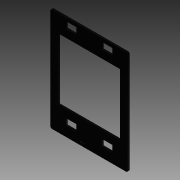
# Autodesk Inventor part: BED HOT BED INSET
Saved by Autodesk Inventor 2013 (Build 170138000, 138)
## iProperties
Created: 2014-03-03
Part Number: BED HOT BED INSET
Material: Generic
Document SubType Name: Modeling
Designer: employee
Density: 1 g/cm^3
Author: employee
Autodesk Inventor part; units mm, degrees
ref_plane "YZ Plane" through (0, 0, 0) normal (1, 0, 0) x (0, 1, 0)
ref_plane "XZ Plane" through (0, 0, 0) normal (0, 1, 0) x (-1, 0, 0)
ref_plane "XY Plane" through (0, 0, 0) normal (0, 0, 1) x (1, 0, 0)
sketch "Sketch1" plane through (0, 0, 0) normal (0, 0, 1) x (1, 0, 0)
  arc A0 (127, -140) -> (122, -135) centre (122, -140) ccw projected
  line L0 (122, -135) -> (119.8284, -135) projected
  line L1 (119.8284, -135) -> (119.8284, -145) projected
  line L2 (119.8284, -145) -> (114.1716, -145) projected
  line L3 (114.1716, -145) -> (114.1716, -135) projected
  line L4 (114.1716, -135) -> (109.5, -135) projected
  arc A1 (107, -132.5) -> (109.5, -135) centre (109.5, -132.5) ccw projected
  line L5 (107, -132.5) -> (107, 132.5) projected
  arc A2 (109.5, 135) -> (107, 132.5) centre (109.5, 132.5) ccw projected
  line L6 (109.5, 135) -> (114.1716, 135) projected
  line L7 (114.1716, 135) -> (114.1716, 145) projected
  line L8 (114.1716, 145) -> (119.8284, 145) projected
  line L9 (119.8284, 145) -> (119.8284, 135) projected
  line L10 (119.8284, 135) -> (122, 135) projected
  arc A3 (122, 135) -> (127, 140) centre (122, 140) ccw projected
  line L11 (127, 140) -> (127, 165) projected
  arc A4 (127, 165) -> (122, 170) centre (122, 165) ccw projected
  line L12 (122, 170) -> (-122, 170) projected
  arc A5 (-122, 170) -> (-127, 165) centre (-122, 165) ccw projected
  line L13 (-127, 165) -> (-127, 140) projected
  arc A6 (-127, 140) -> (-122, 135) centre (-122, 140) ccw projected
  line L14 (-122, 135) -> (-119.8284, 135) projected
  line L15 (-119.8284, 135) -> (-119.8284, 145) projected
  line L16 (-119.8284, 145) -> (-114.1716, 145) projected
  line L17 (-114.1716, 145) -> (-114.1716, 135) projected
  line L18 (-114.1716, 135) -> (-109.5, 135) projected
  arc A7 (-107, 132.5) -> (-109.5, 135) centre (-109.5, 132.5) ccw projected
  line L19 (-107, 132.5) -> (-107, -132.5) projected
  arc A8 (-109.5, -135) -> (-107, -132.5) centre (-109.5, -132.5) ccw projected
  line L20 (-109.5, -135) -> (-114.1716, -135) projected
  line L21 (-114.1716, -135) -> (-114.1716, -145) projected
  line L22 (-114.1716, -145) -> (-119.8284, -145) projected
  line L23 (-119.8284, -145) -> (-119.8284, -135) projected
  line L24 (-119.8284, -135) -> (-122, -135) projected
  arc A9 (-122, -135) -> (-127, -140) centre (-122, -140) ccw projected
  line L25 (-127, -140) -> (-127, -165) projected
  arc A10 (-127, -165) -> (-122, -170) centre (-122, -165) ccw projected
  line L26 (-122, -170) -> (122, -170) projected
  arc A11 (122, -170) -> (127, -165) centre (122, -165) ccw projected
  line L27 (127, -165) -> (127, -140) projected
  line L28 (113, -142) -> (112, -142) projected
  line L29 (112, -142) -> (112, -138) projected
  line L30 (112, -138) -> (113, -138) projected
  line L31 (113, -138) -> (113, -142) projected
  line L32 (121, -142) -> (121, -138) projected
  line L33 (121, -138) -> (122, -138) projected
  line L34 (122, -138) -> (122, -142) projected
  line L35 (122, -142) -> (121, -142) projected
  line L36 (-112, -142) -> (-113, -142) projected
  line L37 (-113, -142) -> (-113, -138) projected
  line L38 (-113, -138) -> (-112, -138) projected
  line L39 (-112, -138) -> (-112, -142) projected
  line L40 (-121, -138) -> (-121, -142) projected
  line L41 (-121, -142) -> (-122, -142) projected
  line L42 (-122, -142) -> (-122, -138) projected
  line L43 (-122, -138) -> (-121, -138) projected
  line L44 (112, 142) -> (113, 142) projected
  line L45 (113, 142) -> (113, 138) projected
  line L46 (113, 138) -> (112, 138) projected
  line L47 (112, 138) -> (112, 142) projected
  line L48 (121, 138) -> (121, 142) projected
  line L49 (121, 142) -> (122, 142) projected
  line L50 (122, 142) -> (122, 138) projected
  line L51 (122, 138) -> (121, 138) projected
  line L52 (-122, 138) -> (-122, 142) projected
  line L53 (-122, 142) -> (-121, 142) projected
  line L54 (-121, 142) -> (-121, 138) projected
  line L55 (-121, 138) -> (-122, 138) projected
  line L56 (-112, 142) -> (-112, 138) projected
  line L57 (-112, 138) -> (-113, 138) projected
  line L58 (-113, 138) -> (-113, 142) projected
  line L59 (-113, 142) -> (-112, 142) projected
  line L60 (-127, 140) -> (-127, -140)
  line L61 (127, -140) -> (127, 140)
  arc A12 (20.5, 83.5) -> (-1.5, 83.5) centre (9.5, 83.5) ccw projected
  line L62 (20.5, 83.5) -> (20.5, -116.5) projected
  arc A13 (-1.5, -116.5) -> (20.5, -116.5) centre (9.5, -116.5) ccw projected
  line L63 (-1.5, -116.5) -> (-1.5, 83.5) projected
  line L64 (42, -96.4) -> (77, -96.4) projected
  line L65 (77, -96.4) -> (77, -138.4) projected
  line L66 (77, -138.4) -> (42, -138.4) projected
  line L67 (42, -138.4) -> (42, -96.4) projected
  line L68 (77, 117.6) -> (42, 117.6) projected
  line L69 (42, 117.6) -> (42, 159.6) projected
  line L70 (42, 159.6) -> (77, 159.6) projected
  line L71 (77, 159.6) -> (77, 117.6) projected
  line L72 (-77, -96.4) -> (-42, -96.4) projected
  line L73 (-42, -96.4) -> (-42, -138.4) projected
  line L74 (-42, -138.4) -> (-77, -138.4) projected
  line L75 (-77, -138.4) -> (-77, -96.4) projected
  line L76 (-42, 117.6) -> (-77, 117.6) projected
  line L77 (-77, 117.6) -> (-77, 159.6) projected
  line L78 (-77, 159.6) -> (-42, 159.6) projected
  line L79 (-42, 159.6) -> (-42, 117.6) projected
  circle A14 centre (0, 165) radius 1.25 projected
  circle A15 centre (0, -165) radius 1.25 projected
  circle A16 centre (-23, -162.38) radius 3.175 projected
  circle A17 centre (-30.6332, -154.7468) radius 0.5 projected
  circle A18 centre (-15.3668, -154.7468) radius 0.5 projected
  point P0 (0, 0)
  constraints: 4 end point, 4 tangent, 1 parallel, 1 perpendicular
extrude "Extrusion1" add sketch "Sketch1" along normal blind 6.477 contours L27 A11 L26 A10 L25 A9 L24 L23 L22 L21 L20 A8 L19 A7 L18 L17 L16 L15 L14 A6 L13 A5 L12 A4 L11 A3 L10 L9 L8 L7 L6 A2 L5 A1 L4 L3 L2 L1 L0 A0 | A0 L0 L1 L2 L3 L4 A1 L5 A2 L6 L7 L8 L9 L10 A3 L61 | L60 A6 L14 L15 L16 L17 L18 A7 L19 A8 L20 L21 L22 L23 L24 A9 | L62 A13 L63 A12 | L64 L65 L66 L67 | L68 L69 L70 L71 | L72 L73 L74 L75 | L76 L77 L78 L79 | A14 | A15 | A16 | A17 | A18
sketch "Sketch2" plane through (0, 0, 6.477) normal (0, 0, 1) x (1, 0, 0)
  line L0 (-122, -170) -> (122, -170) projected
  line L1 (-101.6, 112.2) -> (101.6, 112.2)
  line L2 (101.6, 112.2) -> (101.6, -91)
  line L3 (101.6, -91) -> (-101.6, -91)
  line L4 (-101.6, -91) -> (-101.6, 112.2)
  point P0 (0, 0)
  point P1 (0, -91)
  dimension "d2" = 203.2
  dimension "d4" = 79
  constraints: 8 end point, 2 parallel, 2 perpendicular, 1 horizontal, 1 midpoint, 1 vertical alignment
  measures "d2" distance of L1.end L2.end
  measures "d4" distance between parallel lines of L3 L0
extrude "Extrusion2" cut sketch "Sketch2" against normal through all
sketch "Sketch3" plane through (0, 0, 6.477) normal (0, 0, 1) x (1, 0, 0)
  line L0 (-127, 165) -> (-127, -165) projected
  line L1 (127, 137.6) -> (-127, 137.6) projected
  line L2 (-127, -116.4) -> (127, -116.4) projected
  line L3 (-77, -116.4) -> (-42, -116.4)
  line L4 (-42, -116.4) -> (-42, -138.4)
  line L5 (-42, -138.4) -> (-77, -138.4)
  line L6 (-77, -138.4) -> (-77, -116.4)
  line L7 (77, -116.4) -> (42, -116.4)
  line L8 (42, -116.4) -> (42, -138.4)
  line L9 (42, -138.4) -> (77, -138.4)
  line L10 (77, -138.4) -> (77, -116.4)
  line L11 (-77, 137.6) -> (-42, 137.6)
  line L12 (-42, 137.6) -> (-42, 159.6)
  line L13 (-42, 159.6) -> (-77, 159.6)
  line L14 (-77, 159.6) -> (-77, 137.6)
  line L15 (77, 137.6) -> (42, 137.6)
  line L16 (42, 137.6) -> (42, 159.6)
  line L17 (42, 159.6) -> (77, 159.6)
  line L18 (77, 159.6) -> (77, 137.6)
  line L19 (-42, -138.4) -> (42, -138.4)
  line L20 (-42, 159.6) -> (42, 159.6)
  point P0 (0, 0)
  point P1 (0, -138.4)
  point P2 (0, -116.4)
  point P3 (0, 159.6)
  dimension "d7" = 22
  dimension "d9" = 35
  dimension "d10" = 50
  constraints: 36 end point, 9 parallel, 7 equal length, 5 perpendicular, 4 horizontal, 4 point on line, 3 midpoint, 2 vertical alignment
  measures "d7" distance of L3.end L4.end
  measures "d9" distance of L4.end L5.end
  measures "d10" distance between parallel lines of L6 L0
extrude "Extrusion3" cut sketch "Sketch3" against normal through all contours L2 L4 L5 L6 | L14 L13 L12 L1 | L16 L17 L18 L1 | L2 L10 L9 L8
sketch "Sketch4" plane through (0, 0, 6.477) normal (0, 0, 1) x (1, 0, 0)
  circle A0 centre (0, 165) radius 1.25 projected
  circle A1 centre (0, -165) radius 1.25 projected
  point P0 (0, 0)
extrude "Extrusion4" cut sketch "Sketch4" against normal through all
sketch "Sketch5" plane through (0, 0, 6.477) normal (0, 0, 1) x (1, 0, 0)
  circle A0 centre (-23, -162.38) radius 5.08 projected
  point P0 (0, 0)
extrude "Extrusion5" cut sketch "Sketch5" against normal through all
sketch "Sketch6" plane through (0, 0, 6.477) normal (0, 0, 1) x (1, 0, 0)
  circle A0 centre (-30.6332, -154.7468) radius 0.5 projected
  circle A1 centre (-15.3668, -154.7468) radius 0.5 projected
  circle A2 centre (-23, -162.38) radius 5.08 projected
  line L0 (-15.5, -150) -> (-30.5, -150) projected
  line L1 (-35.5, -155) -> (-35.5, -165) projected
  line L2 (-30.5, -170) -> (-15.5, -170) projected
  line L3 (-10.5, -165) -> (-10.5, -155) projected
  arc A3 (-30.5, -150) -> (-35.5, -155) centre (-30.5, -155) ccw projected
  arc A4 (-35.5, -165) -> (-30.5, -170) centre (-30.5, -165) ccw projected
  arc A5 (-15.5, -170) -> (-10.5, -165) centre (-15.5, -165) ccw projected
  arc A6 (-10.5, -155) -> (-15.5, -150) centre (-15.5, -155) ccw projected
  point P0 (0, 0)
extrude "Extrusion6" cut sketch "Sketch6" against normal through all contours A0 | A1
sketch "Sketch7" plane through (0, 0, 6.477) normal (0, 0, 1) x (1, 0, 0)
  line L0 (-101.6, 112.2) -> (101.6, 112.2) projected
  line L1 (4.7625, 112.2) -> (-4.7625, 112.2)
  line L2 (-4.7625, 112.2) -> (-4.7625, 150.3)
  line L3 (-4.7625, 150.3) -> (4.7625, 150.3)
  line L4 (4.7625, 150.3) -> (4.7625, 112.2)
  point P0 (0, 0)
  point P1 (0, 150.3)
  point P2 (0, 112.2)
  dimension "d19" = 38.1
  dimension "d21" = 9.525
  constraints: 8 end point, 2 midpoint, 2 parallel, 1 horizontal, 1 perpendicular, 1 point on line, 1 vertical alignment
  measures "d19" distance of L3.end L1.start
  measures "d21" distance between parallel lines of L4 L2
extrude "Extrusion7" cut sketch "Sketch7" against normal through all
fillet "Fillet1" radius 4.7625 4 edges at (4.7625, 112.2, 3.2385) (-4.7625, 112.2, 3.2385) (-4.7625, 150.3, 3.2385) (4.7625, 150.3, 3.2385)
body "Solid1"
